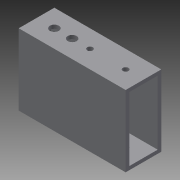
# Autodesk Inventor part: frame_side
Saved by Autodesk Inventor 2015 SP1 (Build 190203100, 203)
## iProperties
Created: 2014-12-22
Part Number: frame_side
Material: Generic
Document SubType Name: Modeling
Designer: Jarod
Density: 1 g/cm^3
Appearance: Default
Author: Jarod
Autodesk Inventor part; units mm, degrees
ref_plane "YZ Plane" through (0, 0, 0) normal (1, 0, 0) x (0, 1, 0)
ref_plane "XZ Plane" through (0, 0, 0) normal (0, 1, 0) x (-1, 0, 0)
ref_plane "XY Plane" through (0, 0, 0) normal (0, 0, 1) x (1, 0, 0)
sketch "Sketch1" plane through (0, 0, 0) normal (1, 0, 0) x (0, 1, 0)
  line L0 (0, 0) -> (50.8, 0)
  line L1 (50.8, 0) -> (50.8, -25.4)
  line L2 (50.8, -25.4) -> (0, -25.4)
  line L3 (0, -25.4) -> (0, 0)
  line L4 (2.54, -2.54) -> (48.26, -2.54)
  line L5 (48.26, -2.54) -> (48.26, -22.86)
  line L6 (48.26, -22.86) -> (2.54, -22.86)
  line L7 (2.54, -22.86) -> (2.54, -2.54)
  dimension "d0" = 50.8
  dimension "d1" = 25.4
  dimension "d2" = 45.72
  dimension "d3" = 20.32
  dimension "d4" = 2.54
  dimension "d5" = 2.54
  constraints: 16 end point, 4 parallel, 2 horizontal, 2 perpendicular
  measures "d0" distance of L1.end L2.end
  measures "d1" distance of L0.end L1.end
  measures "d2" distance of L5.end L6.end
  measures "d3" distance of L4.end L5.end
  measures "d4" distance between parallel lines of L3 L7
  measures "d5" distance between parallel lines of L0 L4
extrude "Extrusion1" add sketch "Sketch1" along normal blind 76.2
sketch "Sketch2" plane through (0, 50.8, 0) normal (0, 1, 0) x (1, 0, 0)
  line L0 (0, 0) -> (0, 25.4) projected
  line L1 (0, 0) -> (76.2, 0) projected
  line L2 (76.2, 25.4) -> (76.2, 0) projected
  line L3 (0, 25.4) -> (76.2, 25.4) projected
  point P0 (12.7, 12.7)
  point P1 (38.1, 12.7)
  point P2 (63.5, 12.7)
  dimension "d8" = 12.7
  dimension "d9" = 12.7
  dimension "d10" = 12.7
  dimension "d11" = 12.7
  dimension "d12" = 38.1
  dimension "d13" = 63.5
  measures "d8" distance from line of L1 point (12.7, 12.7)
  measures "d9" distance from line of L1 point (38.1, 12.7)
  measures "d10" distance from line of L1 point (63.5, 12.7)
  measures "d11" distance from line of L0 point (12.7, 12.7)
  measures "d12" distance from line of L0 point (38.1, 12.7)
  measures "d13" distance from line of L0 point (63.5, 12.7)
hole "Hole1" at (12.7, 50.8, -12.7) at (38.1, 50.8, -12.7) at (63.5, 50.8, -12.7) direction (0, -1, 0) diameter 3.9688 end through all
sketch "Sketch4" plane through (0, 50.8, 0) normal (0, 1, 0) x (1, 0, 0)
  circle A0 centre (38.1, 12.7) radius 1.9844 projected
  circle A1 centre (12.7, 12.7) radius 1.9844 projected
  circle A2 centre (63.5, 12.7) radius 1.9844 projected
  line L0 (0, 0) -> (0, 25.4) projected
  line L1 (0, 0) -> (76.2, 0) projected
  line L2 (76.2, 25.4) -> (76.2, 0) projected
  line L3 (0, 25.4) -> (76.2, 25.4) projected
  circle A3 centre (25.4, 12.7) radius 3.175
  circle A4 centre (12.7, 12.7) radius 3.175
  dimension "d25" = 12.7
  dimension "d26" = 25.4
  dimension "d27" = 6.35
  dimension "d28" = 6.35
  constraints: 2 centre point, 2 coincident
  measures "d25" distance from line of L1 point (25.4, 12.7)
  measures "d26" distance from line of L0 point (25.4, 12.7)
  measures "d27" diameter of A3
  measures "d28" diameter of A4
extrude "Extrusion3" cut sketch "Sketch4" against normal blind 50.8 contours A3 | A4
body "Solid1"
